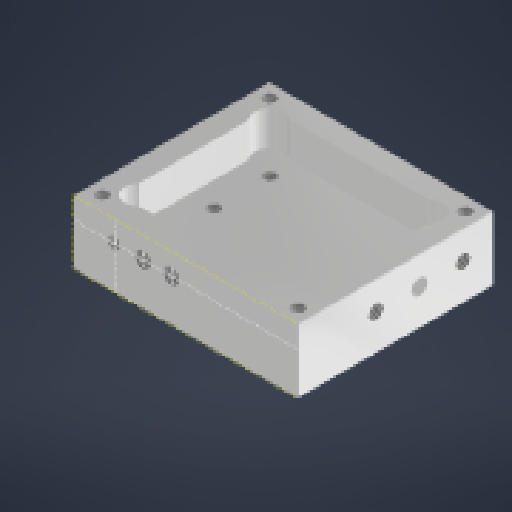
# Autodesk Inventor part: Mixer IQ Box ND20
Saved by Autodesk Inventor 2026.2 (Build 302298010, 298A)
## iProperties
Created: 2009-10-07
Part Number: Mixer IQ Box ND20
Material: Aluminum-6061
Document SubType Name: Modeling
Designer: M. Brock
Mass: 13.5075 g
Surface Area: 35.786 cm^2
Volume: 4.98432 cm^3
Density: 2.71 g/cm^3
Appearance: Aluminum - Flat
Author: M. Brock
Autodesk Inventor part; units mm, degrees
ref_plane "YZ Plane" through (0, 0, 0) normal (1, 0, 0) x (0, 1, 0)
ref_plane "XZ Plane" through (0, 0, 0) normal (0, 1, 0) x (-1, 0, 0)
ref_plane "XY Plane" through (0, 0, 0) normal (0, 0, 1) x (1, 0, 0)
sketch "Sketch1" plane through (0, 0, 0) normal (0, 0, 1) x (1, 0, 0)
  line L0 (0, 0) -> (31.4, 0)
  line L1 (31.4, 0) -> (31.4, 27.4)
  line L2 (31.4, 27.4) -> (0, 27.4)
  line L3 (0, 27.4) -> (0, 0)
  dimension "d0" = 31.4
  dimension "d1" = 27.4
  constraints: 8 end point, 2 parallel, 1 horizontal, 1 perpendicular
  measures "d0" distance between parallel lines of L3 L1
  measures "d1" distance between parallel lines of L2 L0
extrude "Extrusion1" add sketch "Sketch1" along normal blind 4.17
sketch "Sketch2" plane through (0, 0, 4.17) normal (0, 0, 1) x (1, 0, 0)
  line L0 (0, 0) -> (0, 27.4) projected
  line L1 (31.4, 0) -> (0, 0) projected
  line L2 (31.4, 27.4) -> (31.4, 0) projected
  line L3 (0, 27.4) -> (31.4, 27.4) projected
  line L4 (3.2, 3.2) -> (28.2, 3.2)
  line L5 (28.2, 3.2) -> (28.2, 24.2)
  line L6 (28.2, 24.2) -> (3.2, 24.2)
  line L7 (3.2, 24.2) -> (3.2, 3.2)
  line L8 (3.2, 24.2) -> (4.6142, 22.7858)
  line L9 (28.2, 24.2) -> (26.7858, 22.7858)
  line L10 (28.2, 3.2) -> (26.7858, 4.6142)
  line L11 (3.2, 3.2) -> (4.6142, 4.6142)
  circle A0 centre (4.6142, 22.7858) radius 2
  circle A1 centre (26.7858, 22.7858) radius 2
  circle A2 centre (26.7858, 4.6142) radius 2
  circle A3 centre (4.6142, 4.6142) radius 2
  dimension "d11" = 4
  dimension "d12" = 4
  dimension "d13" = 4
  dimension "d14" = 4
  dimension "d4" = 3.2
  dimension "d5" = 3.2
  dimension "d6" = 3.2
  dimension "d8" = 3.2
  dimension "d9" = 45
  dimension "d10" = 45
  constraints: 16 end point, 4 coincident, 3 parallel, 2 perpendicular, 1 horizontal, 12 other
  measures "d4" distance between parallel lines of L1 L4
  measures "d5" distance between parallel lines of L7 L0
  measures "d6" distance between parallel lines of L5 L2
  measures "d8" distance between parallel lines of L6 L3
  measures "d9" angle of L4 L11
  measures "d10" angle of L4 L10
extrude "Extrusion2" add sketch "Sketch2" along normal blind 4.83
sketch "Sketch3" plane through (0, 0, 9) normal (0, 0, 1) x (1, 0, 0)
  line L0 (0, 27.4) -> (31.4, 27.4) projected
  line L1 (0, 0) -> (0, 27.4) projected
  line L2 (31.4, 0) -> (0, 0) projected
  line L3 (31.4, 27.4) -> (31.4, 0) projected
  point P0 (2, 25.4)
  point P1 (29.4, 25.4)
  point P2 (29.4, 2)
  point P3 (2, 2)
  dimension "d17" = 2
  dimension "d18" = 2
  dimension "d19" = 2
  dimension "d20" = 2
  dimension "d21" = 2
  dimension "d22" = 2
  dimension "d23" = 2
  dimension "d24" = 2
  measures "d17" distance from line of L1 point (2, 25.4)
  measures "d18" distance from line of point (2, 25.4) L0
  measures "d19" distance from line of L0 point (29.4, 25.4)
  measures "d20" distance from line of point (29.4, 25.4) L3
  measures "d21" distance from line of point (29.4, 2) L3
  measures "d22" distance from line of point (29.4, 2) L2
  measures "d23" distance from line of point (2, 2) L2
  measures "d24" distance from line of point (2, 2) L1
hole "Hole1" at (2, 25.4, 9) at (29.4, 25.4, 9) at (29.4, 2, 9) at (2, 2, 9) direction (0, 0, -1) diameter 1.6942 end through all thread size "2-56 UNC" class "2B" standard "ANSI Unified Screw Threads"
sketch "Sketch6" plane through (31.4, 0, 0) normal (1, 0, 0) x (0, 0, -1)
  line L0 (0, 0) -> (0, 27.4) projected
  line L1 (0, 27.4) -> (-9, 27.4) projected
  point P0 (-5.06, 17)
  dimension "d50" = 5.06
  dimension "d51" = 10.4
  measures "d50" distance from line of point (-5.06, 17) L0
  measures "d51" distance from line of point (-5.06, 17) L1
hole "Hole4" at (31.4, 17, 5.06) direction (-1, 0, 0) diameter 2.15 depth 3.25
sketch "Sketch7" plane through (31.4, 0, 0) normal (1, 0, 0) x (0, 0, -1)
  circle A0 centre (-5.06, 17) radius 1.075 projected
  line L0 (0, 0) -> (0, 27.4) projected
  point P0 (-5.06, 23.1)
  point P1 (-5.06, 10.9)
  dimension "d59" = 6.1
  dimension "d60" = 6.1
  dimension "d175" = 5.06
  dimension "d176" = 5.06
  measures "d59" distance of point (-5.06, 23.1) A0.centre
  measures "d60" distance of point (-5.06, 10.9) A0.centre
  measures "d175" distance from line of L0 point (-5.06, 23.1)
  measures "d176" distance from line of L0 point (-5.06, 10.9)
hole "Hole5" at (31.4, 23.1, 5.06) at (31.4, 10.9, 5.06) direction (-1, 0, 0) diameter 1.9406 depth 3.5 tip angle 118 thread size "3-48 UNC" class "2B" standard "ANSI Unified Screw Threads"
sketch "Sketch10" plane through (0, 0, 4.17) normal (0, 0, 1) x (1, 0, 0)
  line L0 (0, 27.4) -> (31.4, 27.4) projected
  line L1 (6.6, 20.8) -> (24.8, 20.8) construction
  line L2 (24.8, 20.8) -> (24.8, 13) construction
  line L3 (24.8, 13) -> (6.6, 13) construction
  line L4 (6.6, 13) -> (6.6, 20.8) construction
  line L5 (0, 0) -> (0, 27.4) construction
  dimension "d170" = 6.6
  dimension "d171" = 6.6
  dimension "d172" = 7.8
  dimension "d173" = 18.2
  constraints: 8 end point, 2 coincident, 2 parallel, 1 horizontal, 1 perpendicular
  measures "d170" distance between parallel lines of L5 L4
  measures "d171" distance between parallel lines of L0 L1
  measures "d172" distance of L1.end L2.end
  measures "d173" distance of L2.end L3.end
hole "Hole8" at (6.6, 20.8, 4.17) at (6.6, 13, 4.17) at (24.8, 13, 4.17) at (24.8, 20.8, 4.17) direction (0, 0, -1) diameter 1.6942 depth 3.6 thread size "2-56 UNC" class "2B" standard "ANSI Unified Screw Threads"
sketch "Sketch15" plane through (0, 0, 0) normal (0, -1, 0) x (1, 0, 0)
  line L0 (0, 0) -> (0, 9) construction
  line L1 (0, 6) -> (31.3856, 6) construction
  line L2 (0, 0) -> (31.4, 0) construction
  line L3 (31.4, 9) -> (0, 9) construction
  line L4 (5.7, 9) -> (5.7, 0) construction
  point P0 (9.7, 6)
  point P1 (13.7, 6)
  point P2 (5.7, 6)
  dimension "d133" = 6
  dimension "d136" = 5.7
  dimension "d137" = 4
  dimension "d138" = 8
  constraints: 7 point on line, 4 end point, 2 perpendicular
  measures "d133" distance between parallel lines of L1 L2
  measures "d136" distance between parallel lines of L4 L0
  measures "d137" distance from line of point (9.7, 6) L4
  measures "d138" distance from line of point (13.7, 6) L4
hole "Hole13" at (9.7, 0, 6) at (13.7, 0, 6) direction (0, 1, 0) diameter 2.1565 depth 3.5 tip angle 118 thread size "4-40 UNC" class "2B" standard "ANSI Unified Screw Threads"
hole "Hole15" at (5.7, 0, 6) direction (0, 1, 0) diameter 1.6942 depth 3.5 tip angle 118 thread size "2-56 UNC" class "2B" standard "ANSI Unified Screw Threads"
chamfer "Chamfer1" distance 0.1 angle 45 12 edges at (31.4, 13.7, 9) (15.7, 0, 9) (0, 13.7, 9) (15.7, 27.4, 9) (31.4, 0, 4.5) (31.4, 13.7, 0) (15.7, 0, 0) (31.4, 27.4, 4.5) (15.7, 27.4, 0) (0, 27.4, 4.5) (0, 13.7, 0) (0, 0, 4.5)
equation "\"d12\" = d11"
equation "\"d13\" = d11"
equation "\"d14\" = d11"
equation "\"d5\" = d4"
equation "\"d6\" = d4"
equation "\"d8\" = d4"
equation "\"d10\" = d9"
equation "\"d18\" = d17"
equation "\"d19\" = d17"
equation "\"d20\" = d17"
equation "\"d21\" = d17"
equation "\"d22\" = d17"
equation "\"d23\" = d17"
equation "\"d24\" = d17"
equation "\"d60\" = d59"
body "Solid1"
